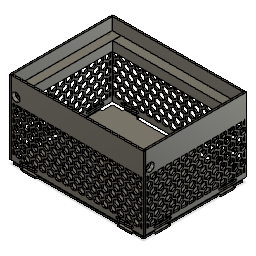
PSVR Storage Cube v1 (Autodesk Fusion 360 design; units mm, degrees)
Autodesk Fusion 360 part; units mm, degrees
(part 1 of 4)
sketch "Sketch1" plane through (0, 0, 0) normal (0, 1, 0) x (1, 0, 0)
  line L0 (0, 0) -> (151, 0)
  line L1 (151, 0) -> (151, 115)
  line L2 (151, 115) -> (0, 115)
  line L3 (0, 115) -> (0, 0)
  dimension "d1" = 151
  dimension "d2" = 115
  constraint horizontal L0
  constraint vertical L1
  constraint horizontal L2
  constraint vertical L3
  constraint coincident L0.start L3.end
  measures "d1" distance of L0.start L0.end
  measures "d2" distance of L0.start L2.end
extrude "Extrude1" add sketch "Sketch1" along normal blind 2 makes body 1
sketch "Sketch2" plane through (0, 0, 0) normal (0, 0, 1) x (1, 0, 0)
  line L0 (-150, 0) -> (1, 0)
  line L1 (1, 0) -> (1, 130)
  line L2 (1, 130) -> (-150, 130)
  line L3 (-150, 130) -> (-150, 0)
  line L4 (-150, 0) -> (1, 0)
  line L5 (1, 0) -> (1, 65)
  line L6 (1, 65) -> (-150, 65)
  line L7 (-150, 65) -> (-150, 0)
  dimension "d5" = 151
  dimension "d6" = 130
  dimension "d14" = 65
  constraint horizontal L0
  constraint vertical L1
  constraint horizontal L2
  constraint vertical L3
  constraint horizontal L4
  constraint vertical L5
  constraint horizontal L6
  constraint vertical L7
  measures "d5" distance of L0.start L0.end
  measures "d6" distance of L0.start L2.end
  measures "d14" distance of L0.start L6.end
extrude "Extrude2" add sketch "Sketch2" along normal blind 2 separate body contours L0 L1 L3 L4 L5 L6 L7 makes body 2
sketch "Sketch3" plane through (0, 0, 0) normal (1, 0, 0) x (0, 0, -1)
  line L0 (200, 0) -> (85, 0)
  line L1 (85, 0) -> (85, 130)
  line L2 (85, 130) -> (200, 130)
  line L3 (200, 130) -> (200, 0)
  line L4 (85, 0) -> (200, 0)
  line L5 (200, 0) -> (200, 65)
  line L6 (200, 65) -> (85, 65)
  line L7 (85, 65) -> (85, 0)
  dimension "d9" = 115
  dimension "d10" = 130
  dimension "d13" = 65
  constraint horizontal L0
  constraint vertical L1
  constraint horizontal L2
  constraint vertical L3
  constraint horizontal L4
  constraint vertical L5
  constraint horizontal L6
  constraint vertical L7
  measures "d9" distance of L0.start L0.end
  measures "d10" distance of L0.start L2.end
  measures "d13" distance of L0.end L6.end
extrude "Extrude3" add sketch "Sketch3" against normal blind 2 separate body contours L0 L1 L3 L4 L5 L6 L7 makes body 3
sketch "Sketch4" plane through (0, 0, 0) normal (1, 0, 0) x (0, 0, -1)
  line L0 (85, 0) -> (200, 0)
  line L1 (200, 0) -> (200, 65)
  line L2 (200, 65) -> (85, 65)
  line L3 (85, 65) -> (85, 0)
  line L4 (200, 0) -> (85, 0)
  line L5 (85, 0) -> (85, 40)
  line L6 (85, 40) -> (200, 40)
  line L7 (200, 40) -> (200, 0)
  line L8 (85, 40) -> (200, 40)
  line L9 (200, 40) -> (200, 51)
  line L10 (200, 51) -> (85, 51)
  line L11 (85, 51) -> (85, 40)
  line L12 (85, 40) -> (95.25, 40)
  line L13 (95.25, 40) -> (95.25, 51)
  line L14 (95.25, 51) -> (85, 51)
  line L15 (85, 51) -> (85, 40)
  dimension "d15" = 40
  dimension "d16" = 11
  dimension "d24" = 10.25
  constraint horizontal L4
  constraint vertical L5
  constraint horizontal L6
  constraint vertical L7
  constraint coincident L0.end L1.start
  constraint horizontal L8
  constraint vertical L9
  constraint horizontal L10
  constraint vertical L11
  constraint horizontal L12
  constraint vertical L13
  constraint horizontal L14
  constraint vertical L15
  measures "d15" distance of L0.end L6.end
  measures "d16" distance of L5.end L10.end
  measures "d24" distance of L5.end L12.end
extrude "Extrude4" add sketch "Sketch4" along normal blind 10 contours L1 L6 L8 L9 L10 L13 bodies 2 3 1
sketch "Sketch5" plane through (0, 0, 0) normal (0, 0, -1) x (-1, 0, 0)
  line L0 (-1, 0) -> (150, 0)
  line L1 (150, 0) -> (150, 65)
  line L2 (150, 65) -> (-1, 65)
  line L3 (-1, 65) -> (-1, 0)
  line L4 (150, 0) -> (-0.75, 0)
  line L5 (-0.75, 0) -> (-0.75, 40)
  line L6 (-0.75, 40) -> (150, 40)
  line L7 (150, 40) -> (150, 0)
  line L8 (-0.75, 40) -> (150, 40)
  line L9 (150, 40) -> (150, 51)
  line L10 (150, 51) -> (-0.75, 51)
  line L11 (-0.75, 51) -> (-0.75, 40)
  line L12 (-0.75, 40) -> (9.25, 40)
  line L13 (9.25, 40) -> (9.25, 51)
  line L14 (9.25, 51) -> (-0.75, 51)
  line L15 (-0.75, 51) -> (-0.75, 40)
  dimension "d19" = 40
  dimension "d20" = 11
  dimension "d23" = 10
  constraint horizontal L4
  constraint vertical L5
  constraint horizontal L6
  constraint vertical L7
  constraint coincident L0.end L1.start
  constraint horizontal L8
  constraint vertical L9
  constraint horizontal L10
  constraint vertical L11
  constraint horizontal L12
  constraint vertical L13
  constraint horizontal L14
  constraint vertical L15
  measures "d19" distance of L0.end L6.end
  measures "d20" distance of L5.end L10.end
  measures "d23" distance of L5.end L12.end
extrude "Extrude5" add sketch "Sketch5" along normal blind 10 contours L1 L6 L8 L9 L10 L13 bodies 3 1 2
extrude "Extrude6" add 1 faces at (-0.6667, 0, -161.6667) along direction (0, -1, 0) blind 20 on bodies 3 bodies 3
extrude "Extrude7" add 1 faces at (-99.6667, 0, 0.6667) along direction (0, -1, 0) blind 20 on bodies 2 bodies 2
move_body "Move1" bodies 2 to x (1, 0, 0) y (0, 1, 0) z (0, 0, 1) at (0, 20, 0)
move_body "Move2" bodies 3 to x (1, 0, 0) y (0, 1, 0) z (0, 0, 1) at (0, 22, 0)
move_body "Move3" bodies 2 to x (1, 0, 0) y (0, 1, 0) z (0, 0, 1) at (150, 0, 0)
move_body "Move4" bodies 3 to x (1, 0, 0) y (0, 1, 0) z (0, 0, 1) at (0, 0, 85)
move_body "Move5" bodies 3 to x (1, 0, 0) y (0, 1, 0) z (0, 0, 1) at (0, -2, 0)
extrude "Extrude8" add 1 faces at (151, 28.3333, 1.3333) along direction (1, 0, 0) blind 2 on bodies 2 bodies 2
extrude "Extrude9" add 1 faces at (-1.3333, 28.3333, 0) along direction (0, 0, 1) blind 2 on bodies 3 bodies 3
sketch "Sketch6" plane through (0, 0, 0) normal (0, 0, -1) x (-1, 0, 0)
  line L0 (-140.75, 71) -> (0, 71)
  line L1 (0, 71) -> (0, 85)
  line L2 (0, 85) -> (-153, 85)
  line L3 (-153, 85) -> (-153, 0)
  line L4 (-153, 0) -> (0, 0)
  line L5 (0, 0) -> (0, 60)
  line L6 (0, 60) -> (-140.75, 60)
  line L7 (-140.75, 60) -> (-140.75, 71)
  line L8 (-153, 0) -> (-141, 0)
  line L9 (-141, 0) -> (-141, 2)
  line L10 (-141, 2) -> (-153, 2)
  line L11 (-153, 2) -> (-153, 0)
  line L12 (-141, 2) -> (-121, 2)
  line L13 (-121, 2) -> (-121, 4.5)
  line L14 (-121, 4.5) -> (-141, 4.5)
  line L15 (-141, 4.5) -> (-141, 2)
  line L16 (0, 0) -> (-10, 0)
  line L17 (-10, 0) -> (-10, 2)
  line L18 (-10, 2) -> (0, 2)
  line L19 (0, 2) -> (0, 0)
  line L20 (-10, 2) -> (-30, 2)
  line L21 (-30, 2) -> (-30, 4.5)
  line L22 (-30, 4.5) -> (-10, 4.5)
  line L23 (-10, 4.5) -> (-10, 2)
  dimension "d33" = 12
  dimension "d34" = 2
  dimension "d35" = 20
  dimension "d36" = 2.5
  dimension "d37" = 10
  dimension "d38" = 2
  dimension "d39" = 20
  dimension "d40" = 2.5
  constraint horizontal L8
  constraint vertical L9
  constraint horizontal L10
  constraint vertical L11
  constraint coincident L3.end L4.start
  constraint horizontal L12
  constraint vertical L13
  constraint horizontal L14
  constraint vertical L15
  constraint horizontal L16
  constraint vertical L17
  constraint horizontal L18
  constraint vertical L19
  constraint coincident L4.end L5.start
  constraint horizontal L20
  constraint vertical L21
  constraint horizontal L22
  constraint vertical L23
  measures "d33" distance of L3.end L8.end
  measures "d34" distance of L3.end L10.end
  measures "d35" distance of L9.end L12.end
  measures "d36" distance of L9.end L14.end
  measures "d37" distance of L4.end L16.end
  measures "d38" distance of L4.end L18.end
  measures "d39" distance of L17.end L20.end
  measures "d40" distance of L17.end L22.end
extrude "Extrude10" cut sketch "Sketch6" against normal blind 2 contours L12 L13 L14 L15 | L20 L21 L22 L23 bodies 2
sketch "Sketch7" plane through (0, 0, 0) normal (1, 0, 0) x (0, 0, -1)
  line L0 (10.25, 71) -> (115, 71)
  line L1 (115, 71) -> (115, 85)
  line L2 (115, 85) -> (-2, 85)
  line L3 (-2, 85) -> (-2, 0)
  line L4 (-2, 0) -> (115, 0)
  line L5 (115, 0) -> (115, 60)
  line L6 (115, 60) -> (10.25, 60)
  line L7 (10.25, 60) -> (10.25, 71)
  line L8 (-2, 0) -> (10, 0)
  line L9 (10, 0) -> (10, 2)
  line L10 (10, 2) -> (-2, 2)
  line L11 (-2, 2) -> (-2, 0)
  line L12 (10, 2) -> (30, 2)
  line L13 (30, 2) -> (30, 4.5)
  line L14 (30, 4.5) -> (10, 4.5)
  line L15 (10, 4.5) -> (10, 2)
  line L16 (115, 0) -> (105, 0)
  line L17 (105, 0) -> (105, 2)
  line L18 (105, 2) -> (115, 2)
  line L19 (115, 2) -> (115, 0)
  line L20 (105, 2) -> (85, 2)
  line L21 (85, 2) -> (85, 4.5)
  line L22 (85, 4.5) -> (105, 4.5)
  line L23 (105, 4.5) -> (105, 2)
  dimension "d43" = 12
  dimension "d44" = 2
  dimension "d45" = 20
  dimension "d46" = 2.5
  dimension "d47" = 10
  dimension "d48" = 2
  dimension "d49" = 20
  dimension "d50" = 2.5
  constraint horizontal L8
  constraint vertical L9
  constraint horizontal L10
  constraint vertical L11
  constraint coincident L3.end L4.start
  constraint horizontal L12
  constraint vertical L13
  constraint horizontal L14
  constraint vertical L15
  constraint horizontal L16
  constraint vertical L17
  constraint horizontal L18
  constraint vertical L19
  constraint coincident L4.end L5.start
  constraint horizontal L20
  constraint vertical L21
  constraint horizontal L22
  constraint vertical L23
  measures "d43" distance of L3.end L8.end
  measures "d44" distance of L3.end L10.end
  measures "d45" distance of L9.end L12.end
  measures "d46" distance of L9.end L14.end
  measures "d47" distance of L4.end L16.end
  measures "d48" distance of L4.end L18.end
  measures "d49" distance of L17.end L20.end
  measures "d50" distance of L17.end L22.end
extrude "Extrude11" cut sketch "Sketch7" against normal blind 2 contours L12 L13 L14 L15 | L20 L21 L22 L23 bodies 3
move_body "Move6" bodies 1 to x (1, 0, 0) y (0, 1, 0) z (0, 0, 1) at (0, -5, 0)
sketch "Sketch8" plane through (0, -3, 0) normal (0, 1, 0) x (-1, 0, 0)
  line L0 (0, -115) -> (0, 0)
  line L1 (0, 0) -> (-151, 0)
  line L2 (-151, 0) -> (-151, -115)
  line L3 (-151, -115) -> (0, -115)
  line L4 (0, -115) -> (-20, -115)
  line L5 (-20, -115) -> (-29, -115)
  line L6 (-29, -115) -> (-11, -115)
  line L7 (-11, -115) -> (-11, -117)
  line L8 (-11, -117) -> (-29, -117)
  line L9 (-29, -117) -> (-29, -115)
  line L10 (-151, -115) -> (-122, -115)
  line L11 (-122, -115) -> (-140, -115)
  line L12 (-140, -115) -> (-140, -117)
  line L13 (-140, -117) -> (-122, -117)
  line L14 (-122, -117) -> (-122, -115)
  line L15 (0, -115) -> (0, -86)
  line L16 (0, -86) -> (2, -86)
  line L17 (2, -86) -> (2, -104)
  line L18 (2, -104) -> (0, -104)
  line L19 (0, -104) -> (0, -86)
  line L20 (-151, -115) -> (-151, -86)
  line L21 (-151, -86) -> (-153, -86)
  line L22 (-153, -86) -> (-153, -104)
  line L23 (-153, -104) -> (-151, -104)
  line L24 (-151, -104) -> (-151, -86)
  line L25 (-151, 0) -> (-122, 0)
  line L26 (-122, 0) -> (-140, 0)
  line L27 (-140, 0) -> (-140, 2)
  line L28 (-140, 2) -> (-122, 2)
  line L29 (-122, 2) -> (-122, 0)
  line L30 (-151, 0) -> (-151, -29)
  line L31 (-151, -29) -> (-153, -29)
  line L32 (-153, -29) -> (-153, -11)
  line L33 (-153, -11) -> (-151, -11)
  line L34 (-151, -11) -> (-151, -29)
  line L35 (0, 0) -> (-29, 0)
  line L36 (-29, 0) -> (-11, 0)
  line L37 (-11, 0) -> (-11, 2)
  line L38 (-11, 2) -> (-29, 2)
  line L39 (-29, 2) -> (-29, 0)
  line L40 (0, 0) -> (0, -29)
  line L41 (0, -29) -> (2, -29)
  line L42 (2, -29) -> (2, -11)
  line L43 (2, -11) -> (0, -11)
  line L44 (0, -11) -> (0, -29)
  dimension "d53" = 20
  dimension "d54" = 9
  dimension "d55" = 18
  dimension "d56" = 2
  dimension "d57" = 29
  dimension "d58" = 18
  dimension "d59" = 2
  dimension "d60" = 29
  dimension "d61" = 2
  dimension "d62" = 18
  dimension "d63" = 29
  dimension "d64" = 2
  dimension "d65" = 18
  dimension "d66" = 29
  dimension "d67" = 18
  dimension "d68" = 2
  dimension "d69" = 29
  dimension "d70" = 2
  dimension "d71" = 18
  dimension "d72" = 29
  dimension "d73" = 18
  dimension "d74" = 2
  dimension "d75" = 29
  dimension "d76" = 2
  dimension "d77" = 18
  constraint coincident L0.start L3.end
  constraint perpendicular L0 L4
  constraint parallel L3 L5
  constraint horizontal L6
  constraint vertical L7
  constraint horizontal L8
  constraint vertical L9
  constraint coincident L2.end L3.start
  constraint perpendicular L2 L10
  constraint horizontal L11
  constraint vertical L12
  constraint horizontal L13
  constraint vertical L14
  constraint perpendicular L4 L15
  constraint horizontal L16
  constraint vertical L17
  constraint horizontal L18
  constraint vertical L19
  constraint perpendicular L10 L20
  constraint horizontal L21
  constraint vertical L22
  constraint horizontal L23
  constraint vertical L24
  constraint coincident L1.end L2.start
  constraint perpendicular L2 L25
  constraint horizontal L26
  constraint vertical L27
  constraint horizontal L28
  constraint vertical L29
  constraint perpendicular L1 L30
  constraint horizontal L31
  constraint vertical L32
  constraint horizontal L33
  constraint vertical L34
  constraint coincident L0.end L1.start
  constraint perpendicular L0 L35
  constraint horizontal L36
  constraint vertical L37
  constraint horizontal L38
  constraint vertical L39
  constraint perpendicular L35 L40
  constraint horizontal L41
  constraint vertical L42
  constraint horizontal L43
  constraint vertical L44
  measures "d53" distance of L0.start L4.end
  measures "d54" distance of L4.end L5.end
  measures "d55" distance of L5.end L6.end
  measures "d56" distance of L5.end L8.end
  measures "d57" distance of L2.end L10.end
  measures "d58" distance of L10.end L11.end
  measures "d59" distance of L10.end L13.end
  measures "d60" distance of L0.start L15.end
  measures "d61" distance of L15.end L16.end
  measures "d62" distance of L15.end L18.end
  measures "d63" distance of L2.end L20.end
  measures "d64" distance of L20.end L21.end
  measures "d65" distance of L20.end L23.end
  measures "d66" distance of L1.end L25.end
  measures "d67" distance of L25.end L26.end
  measures "d68" distance of L25.end L28.end
  measures "d69" distance of L1.end L30.end
  measures "d70" distance of L30.end L31.end
  measures "d71" distance of L30.end L33.end
  measures "d72" distance of L0.end L35.end
  measures "d73" distance of L35.end L36.end
  measures "d74" distance of L35.end L38.end
  measures "d75" distance of L0.end L40.end
  measures "d76" distance of L40.end L41.end
  measures "d77" distance of L40.end L43.end
extrude "Extrude12" add sketch "Sketch8" against normal blind 2 contours L0 L15 L16 L17 L18 L19 | L3 L4 L5 L6 L7 L8 L9 | L0 L40 L41 L42 L43 L44 | L3 L10 L11 L12 L13 L14 | L1 L35 L36 L37 L38 L39 | L2 L20 L21 L22 L23 L24 | L1 L25 L26 L27 L28 L29 | L2 L30 L31 L32 L33 L34 bodies 1
fillet "Fillet1" radius 1 32 edges at (-1, -3, -11) (-1, -5, -11) (-1, -5, -29) (-1, -3, -29) (-1, -3, -104) (-1, -5, -104) (-1, -5, -86) (-1, -3, -86) (11, -3, -116) (11, -5, -116) (29, -3, -116) (29, -5, -116) (122, -3, -116) (140, -3, -116) (140, -5, -116) (152, -3, -104) (152, -5, -104) (152, -3, -86) (122, -5, -116) (152, -5, -86) (152, -3, -29) (152, -5, -29) (152, -3, -11) (152, -5, -11) (140, -5, 1) (140, -3, 1) (122, -5, 1) (122, -3, 1) (29, -3, 1) (29, -5, 1) (11, -3, 1) (11, -5, 1) on bodies 1
fillet "Fillet2" radius 1 16 edges at (141, 4.5, 1) (141, 2, 1) (30, 2, 1) (10, 2, 1) (10, 4.5, 1) (30, 4.5, 1) (121, 2, 1) (121, 4.5, 1) (-1, 4.5, -85) (-1, 4.5, -10) (-1, 2, -85) (-1, 2, -10) (-1, 4.5, -30) (-1, 2, -30) (-1, 2, -105) (-1, 4.5, -105) on bodies 2 3
move_face "OffsetFaces1" offset -0.25 12 faces at (151, -3.9049, -48) (151, -4.0001, -111.3333) (147.3333, -4.0001, -115) (91, -4.1159, -115) (151, -4.0001, -3.6667) (147.3333, -3.9999, 0) (60, -4.1159, 0) (3.6667, -4.0001, 0) (0, -4.0001, -3.6667) (0, -3.9049, -67) (0, -4.0001, -111.3333) (3.6667, -3.9999, -115) on bodies 1
sketch "Sketch9" plane through (0, 0, 0) normal (0, 0, -1) x (-1, 0, 0)
  line L0 (-30, 3) -> (-30, 3.5)
  arc A0 (-29, 4.5) -> (-30, 3.5) centre (-29, 3.5) ccw
  line L1 (-29, 4.5) -> (-11, 4.5)
  arc A1 (-10, 3.5) -> (-11, 4.5) centre (-11, 3.5) ccw
  line L2 (-10, 3.5) -> (-10, 3)
  arc A2 (-11, 2) -> (-10, 3) centre (-11, 3) ccw
  line L3 (-11, 2) -> (-29, 2)
  arc A3 (-30, 3) -> (-29, 2) centre (-29, 3) ccw
  line L4 (-122, 2) -> (-140, 2)
  arc A4 (-141, 3) -> (-140, 2) centre (-140, 3) ccw
  line L5 (-141, 3) -> (-141, 3.5)
  arc A5 (-140, 4.5) -> (-141, 3.5) centre (-140, 3.5) ccw
  line L6 (-140, 4.5) -> (-122, 4.5)
  arc A6 (-121, 3.5) -> (-122, 4.5) centre (-122, 3.5) ccw
  line L7 (-121, 3.5) -> (-121, 3)
  arc A7 (-122, 2) -> (-121, 3) centre (-122, 3) ccw
  line L8 (-140.75, 71) -> (0, 71)
  line L9 (0, 71) -> (0, 85)
  line L10 (0, 85) -> (-153, 85)
  line L11 (-153, 85) -> (-153, 0)
  line L12 (-153, 0) -> (0, 0)
  line L13 (0, 0) -> (0, 60)
  line L14 (0, 60) -> (-140.75, 60)
  line L15 (-140.75, 60) -> (-140.75, 71)
  line L16 (0, 60) -> (0, 71)
  line L17 (0, 65.5) -> (-5.5, 65.5)
  circle A8 centre (-5.5, 65.5) radius 4.75
  dimension "d85" = 5.5
  dimension "d86" = 9.5
  constraint coincident L13.end L14.start
  constraint coincident L8.end L9.start
  constraint midpoint L16 L17.start
  constraint perpendicular L16 L17
  constraint coincident L17.end A8.centre
  measures "d85" distance of L17.start L17.end
  measures "d86" diameter of A8
extrude "Extrude13" cut sketch "Sketch9" along normal blind 2 and the other way blind 2 contours A8 bodies 2
sketch "Sketch10" plane through (0, 0, -2) normal (0, 0, 1) x (1, 0, 0)
  circle A0 centre (5.5, 65.5) radius 4.75
  circle A1 centre (5.5, 65.5) radius 2.4
  dimension "d91" = 4.8
  constraint concentric A0 A1
  measures "d91" diameter of A1
extrude "Extrude14" cut sketch "Sketch10" against normal blind 25 contours A1 bodies 2 3
move_face "OffsetFaces2" offset -0.25 1 faces at (0, 67.3333, -6.6667) on bodies 2
sketch "Sketch11" plane through (0, 0, 0) normal (1, 0, 0) x (0, 0, -1)
  line L0 (85, 3) -> (85, 3.5)
  arc A0 (86, 4.5) -> (85, 3.5) centre (86, 3.5) ccw
  line L1 (86, 4.5) -> (104, 4.5)
  arc A1 (105, 3.5) -> (104, 4.5) centre (104, 3.5) ccw
  line L2 (105, 3.5) -> (105, 3)
  arc A2 (104, 2) -> (105, 3) centre (104, 3) ccw
  line L3 (104, 2) -> (86, 2)
  arc A3 (85, 3) -> (86, 2) centre (86, 3) ccw
  line L4 (29, 2) -> (11, 2)
  arc A4 (10, 3) -> (11, 2) centre (11, 3) ccw
  line L5 (10, 3) -> (10, 3.5)
  arc A5 (11, 4.5) -> (10, 3.5) centre (11, 3.5) ccw
  line L6 (11, 4.5) -> (29, 4.5)
  arc A6 (30, 3.5) -> (29, 4.5) centre (29, 3.5) ccw
  line L7 (30, 3.5) -> (30, 3)
  arc A7 (29, 2) -> (30, 3) centre (29, 3) ccw
  line L8 (10.25, 71) -> (115, 71)
  line L9 (115, 71) -> (115, 85)
  line L10 (115, 85) -> (-2, 85)
  line L11 (-2, 85) -> (-2, 0)
  line L12 (-2, 0) -> (115, 0)
  line L13 (115, 0) -> (115, 60)
  line L14 (115, 60) -> (10.25, 60)
  line L15 (10.25, 60) -> (10.25, 71)
  line L16 (115, 60) -> (115, 71)
  line L17 (115, 65.5) -> (109.5, 65.5)
  circle A8 centre (109.5, 65.5) radius 4.75
  dimension "d95" = 5.5
  dimension "d96" = 9.5
  constraint coincident L13.end L14.start
  constraint coincident L8.end L9.start
  constraint midpoint L16 L17.start
  constraint perpendicular L16 L17
  constraint coincident L17.end A8.centre
  measures "d95" distance of L17.start L17.end
  measures "d96" diameter of A8
extrude "Extrude15" cut sketch "Sketch11" along normal blind 2 and the other way blind 2 contours A8 bodies 3
sketch "Sketch12" plane through (2, 0, 0) normal (-1, 0, 0) x (0, 0, 1)
  circle A0 centre (-109.5, 65.5) radius 4.75
  circle A1 centre (-109.5, 65.5) radius 2.4
  dimension "d101" = 4.8
  constraint concentric A0 A1
  measures "d101" diameter of A1
extrude "Extrude16" cut sketch "Sketch12" against normal blind 33 contours A1 bodies 3
sketch "Sketch13" plane through (140.75, 0, 0) normal (1, 0, 0) x (0, 0, -1)
  line L0 (0, 71) -> (0, 60)
  line L1 (0, 60) -> (10, 60)
  line L2 (10, 60) -> (10, 71)
  line L3 (10, 71) -> (0, 71)
  line L4 (10, 65.5) -> (7.9, 65.5)
  circle A0 centre (5.5, 65.5) radius 2.4
  dimension "d104" = 2.1
  dimension "d105" = 4.8
  constraint midpoint L2 L4.start
  constraint perpendicular L2 L4
  constraint coincident L4.end A0
  measures "d104" distance of L4.start L4.end
  measures "d105" diameter of A0
extrude "Extrude17" cut sketch "Sketch13" against normal blind 16.75 contours A0 bodies 2
move_face "OffsetFaces3" offset -0.25 1 faces at (6.6667, 67.3333, -115) on bodies 3
sketch "Sketch14" plane through (0, 0, 0) normal (0, 0, -1) x (-1, 0, 0)
  line L0 (-30, 3) -> (-30, 3.5)
  arc A0 (-29, 4.5) -> (-30, 3.5) centre (-29, 3.5) ccw
  line L1 (-29, 4.5) -> (-11, 4.5)
  arc A1 (-10, 3.5) -> (-11, 4.5) centre (-11, 3.5) ccw
  line L2 (-10, 3.5) -> (-10, 3)
  arc A2 (-11, 2) -> (-10, 3) centre (-11, 3) ccw
  line L3 (-11, 2) -> (-29, 2)
  arc A3 (-30, 3) -> (-29, 2) centre (-29, 3) ccw
  line L4 (-122, 2) -> (-140, 2)
  arc A4 (-141, 3) -> (-140, 2) centre (-140, 3) ccw
  line L5 (-141, 3) -> (-141, 3.5)
  arc A5 (-140, 4.5) -> (-141, 3.5) centre (-140, 3.5) ccw
  line L6 (-140, 4.5) -> (-122, 4.5)
  arc A6 (-121, 3.5) -> (-122, 4.5) centre (-122, 3.5) ccw
  line L7 (-121, 3.5) -> (-121, 3)
  arc A7 (-122, 2) -> (-121, 3) centre (-122, 3) ccw
  line L8 (-140.75, 71) -> (-0.25, 71)
  line L9 (-0.25, 71) -> (-0.25, 85)
  line L10 (-0.25, 85) -> (-153, 85)
  line L11 (-153, 85) -> (-153, 0)
  line L12 (-153, 0) -> (-0.25, 0)
  line L13 (-0.25, 0) -> (-0.25, 60)
  line L14 (-0.25, 60) -> (-140.75, 60)
  line L15 (-140.75, 60) -> (-140.75, 71)
  line L16 (-153, 0) -> (-0.25, 0)
  line L17 (-0.25, 0) -> (-0.25, 6.5)
  line L18 (-0.25, 6.5) -> (-2.25, 6.5)
  line L19 (-2.25, 6.5) -> (-2.25, 85)
  line L20 (-2.25, 85) -> (-0.25, 85)
  line L21 (-0.25, 85) -> (-0.25, 6.5)
  line L22 (-2.25, 85) -> (-153, 85)
  line L23 (-153, 85) -> (-153, 83)
  line L24 (-153, 83) -> (-2.25, 83)
  line L25 (-2.25, 83) -> (-2.25, 85)
  line L26 (-153, 83) -> (-151, 83)
  line L27 (-151, 83) -> (-151, 6.5)
  line L28 (-153, 6.5) -> (-153, 83)
  line L29 (-2.25, 6.5) -> (-2.25, 60)
  line L30 (-2.25, 60) -> (-151, 60)
  line L31 (-151, 60) -> (-151, 6.5)
  line L32 (-153, 0) -> (-0.25, 0)
  line L33 (-0.25, 0) -> (-0.25, 7)
  line L34 (-0.25, 7) -> (-0.25, 0)
  line L35 (-0.25, 0) -> (-153, 0)
  line L36 (-153, 0) -> (-2.25, 0)
  line L37 (-2.25, 0) -> (-2.25, 6)
  line L38 (-2.25, 6) -> (-153, 6)
  line L39 (-153, 6) -> (-153, 0)
  line L40 (-151, 6.5) -> (-151, 6)
  line L41 (-73.125, 35.2707) -> (-76.625, 37.2915)
  line L42 (-76.625, 37.2915) -> (-80.125, 35.2707)
  line L43 (-80.125, 35.2707) -> (-80.125, 31.2293)
  line L44 (-80.125, 31.2293) -> (-76.625, 29.2085)
  line L45 (-76.625, 29.2085) -> (-73.125, 31.2293)
  line L46 (-73.125, 31.2293) -> (-73.125, 35.2707)
  line L47 (-64.125, 35.2707) -> (-67.625, 37.2915)
  line L48 (-67.625, 37.2915) -> (-71.125, 35.2707)
  line L49 (-71.125, 35.2707) -> (-71.125, 31.2293)
  line L50 (-71.125, 31.2293) -> (-67.625, 29.2085)
  line L51 (-67.625, 29.2085) -> (-64.125, 31.2293)
  line L52 (-64.125, 31.2293) -> (-64.125, 35.2707)
  line L53 (-68.625, 43.065) -> (-72.125, 45.0857)
  line L54 (-72.125, 45.0857) -> (-75.625, 43.065)
  line L55 (-75.625, 43.065) -> (-75.625, 39.0235)
  line L56 (-75.625, 39.0235) -> (-72.125, 37.0028)
  line L57 (-72.125, 37.0028) -> (-68.625, 39.0235)
  line L58 (-68.625, 39.0235) -> (-68.625, 43.065)
  line L59 (-77.625, 43.065) -> (-81.125, 45.0857)
  line L60 (-81.125, 45.0857) -> (-84.625, 43.065)
  line L61 (-84.625, 43.065) -> (-84.625, 39.0235)
  line L62 (-84.625, 39.0235) -> (-81.125, 37.0028)
  line L63 (-81.125, 37.0028) -> (-77.625, 39.0235)
  line L64 (-77.625, 39.0235) -> (-77.625, 43.065)
  line L65 (-140.625, 11.311) -> (-144.125, 13.3317)
  line L66 (-144.125, 13.3317) -> (-147.625, 11.311)
  line L67 (-140.625, 7.2695) -> (-140.625, 11.311)
  line L68 (-152.125, 3.5167) -> (-152.125, -0.5247)
  line L69 (-145.125, -0.5247) -> (-145.125, 3.5167)
  line L70 (-147.625, 7.2695) -> (-144.125, 5.2488)
  line L71 (-153.125, 13.3317) -> (-156.625, 11.311)
  line L72 (-149.625, 7.2695) -> (-149.625, 11.311)
  line L73 (-148.625, 5.5375) -> (-152.125, 3.5167)
  line L74 (-148.625, -2.5455) -> (-145.125, -0.5247)
  line L75 (-149.625, 11.311) -> (-153.125, 13.3317)
  line L76 (-156.625, 7.2695) -> (-153.125, 5.2488)
  line L77 (-153.125, 5.2488) -> (-149.625, 7.2695)
  line L78 (-145.125, 3.5167) -> (-148.625, 5.5375)
  line L79 (-147.625, 11.311) -> (-147.625, 7.2695)
  line L80 (-156.625, 11.311) -> (-156.625, 7.2695)
  line L81 (-144.125, 5.2488) -> (-140.625, 7.2695)
  line L82 (-139.625, 5.5375) -> (-143.125, 3.5167)
  line L83 (-136.125, 3.5167) -> (-139.625, 5.5375)
  line L84 (-139.625, -2.5455) -> (-136.125, -0.5247)
  line L85 (-143.125, 3.5167) -> (-143.125, -0.5247)
  line L86 (-143.125, -0.5247) -> (-139.625, -2.5455)
  line L87 (-136.125, -0.5247) -> (-136.125, 3.5167)
  line L88 (-152.125, -0.5247) -> (-148.625, -2.5455)
  line L89 (-122.625, 11.311) -> (-126.125, 13.3317)
  line L90 (-126.125, 13.3317) -> (-129.625, 11.311)
  line L91 (-122.625, 7.2695) -> (-122.625, 11.311)
  line L92 (-134.125, 3.5167) -> (-134.125, -0.5247)
  line L93 (-127.125, -0.5247) -> (-127.125, 3.5167)
  line L94 (-129.625, 7.2695) -> (-126.125, 5.2488)
  line L95 (-135.125, 13.3317) -> (-138.625, 11.311)
  line L96 (-131.625, 7.2695) -> (-131.625, 11.311)
  line L97 (-130.625, 5.5375) -> (-134.125, 3.5167)
  line L98 (-130.625, -2.5455) -> (-127.125, -0.5247)
  line L99 (-131.625, 11.311) -> (-135.125, 13.3317)
  line L100 (-138.625, 7.2695) -> (-135.125, 5.2488)
  line L101 (-135.125, 5.2488) -> (-131.625, 7.2695)
  line L102 (-127.125, 3.5167) -> (-130.625, 5.5375)
  line L103 (-129.625, 11.311) -> (-129.625, 7.2695)
  line L104 (-138.625, 11.311) -> (-138.625, 7.2695)
  line L105 (-126.125, 5.2488) -> (-122.625, 7.2695)
  line L106 (-121.625, 5.5375) -> (-125.125, 3.5167)
  line L107 (-118.125, 3.5167) -> (-121.625, 5.5375)
  line L108 (-121.625, -2.5455) -> (-118.125, -0.5247)
  line L109 (-125.125, 3.5167) -> (-125.125, -0.5247)
  line L110 (-125.125, -0.5247) -> (-121.625, -2.5455)
  line L111 (-118.125, -0.5247) -> (-118.125, 3.5167)
  line L112 (-134.125, -0.5247) -> (-130.625, -2.5455)
  line L113 (-104.625, 11.311) -> (-108.125, 13.3317)
  line L114 (-108.125, 13.3317) -> (-111.625, 11.311)
  line L115 (-104.625, 7.2695) -> (-104.625, 11.311)
  line L116 (-116.125, 3.5167) -> (-116.125, -0.5247)
  line L117 (-109.125, -0.5247) -> (-109.125, 3.5167)
  line L118 (-111.625, 7.2695) -> (-108.125, 5.2488)
  line L119 (-117.125, 13.3317) -> (-120.625, 11.311)
  line L120 (-113.625, 7.2695) -> (-113.625, 11.311)
  line L121 (-112.625, 5.5375) -> (-116.125, 3.5167)
  line L122 (-112.625, -2.5455) -> (-109.125, -0.5247)
  line L123 (-113.625, 11.311) -> (-117.125, 13.3317)
  line L124 (-120.625, 7.2695) -> (-117.125, 5.2488)
  line L125 (-117.125, 5.2488) -> (-113.625, 7.2695)
  line L126 (-109.125, 3.5167) -> (-112.625, 5.5375)
  line L127 (-111.625, 11.311) -> (-111.625, 7.2695)
  line L128 (-120.625, 11.311) -> (-120.625, 7.2695)
  line L129 (-108.125, 5.2488) -> (-104.625, 7.2695)
  line L130 (-103.625, 5.5375) -> (-107.125, 3.5167)
  line L131 (-100.125, 3.5167) -> (-103.625, 5.5375)
  line L132 (-103.625, -2.5455) -> (-100.125, -0.5247)
  line L133 (-107.125, 3.5167) -> (-107.125, -0.5247)
  line L134 (-107.125, -0.5247) -> (-103.625, -2.5455)
  line L135 (-100.125, -0.5247) -> (-100.125, 3.5167)
  line L136 (-116.125, -0.5247) -> (-112.625, -2.5455)
  line L137 (-86.625, 11.311) -> (-90.125, 13.3317)
  line L138 (-90.125, 13.3317) -> (-93.625, 11.311)
  line L139 (-86.625, 7.2695) -> (-86.625, 11.311)
  line L140 (-98.125, 3.5167) -> (-98.125, -0.5247)
  line L141 (-91.125, -0.5247) -> (-91.125, 3.5167)
  line L142 (-93.625, 7.2695) -> (-90.125, 5.2488)
  line L143 (-99.125, 13.3317) -> (-102.625, 11.311)
  line L144 (-95.625, 7.2695) -> (-95.625, 11.311)
  line L145 (-94.625, 5.5375) -> (-98.125, 3.5167)
  line L146 (-94.625, -2.5455) -> (-91.125, -0.5247)
  line L147 (-95.625, 11.311) -> (-99.125, 13.3317)
  line L148 (-102.625, 7.2695) -> (-99.125, 5.2488)
  line L149 (-99.125, 5.2488) -> (-95.625, 7.2695)
  line L150 (-91.125, 3.5167) -> (-94.625, 5.5375)
  line L151 (-93.625, 11.311) -> (-93.625, 7.2695)
  line L152 (-102.625, 11.311) -> (-102.625, 7.2695)
  line L153 (-90.125, 5.2488) -> (-86.625, 7.2695)
  line L154 (-85.625, 5.5375) -> (-89.125, 3.5167)
  line L155 (-82.125, 3.5167) -> (-85.625, 5.5375)
  line L156 (-85.625, -2.5455) -> (-82.125, -0.5247)
  line L157 (-89.125, 3.5167) -> (-89.125, -0.5247)
  line L158 (-89.125, -0.5247) -> (-85.625, -2.5455)
  line L159 (-82.125, -0.5247) -> (-82.125, 3.5167)
  line L160 (-98.125, -0.5247) -> (-94.625, -2.5455)
  line L161 (-68.625, 11.311) -> (-72.125, 13.3317)
  line L162 (-72.125, 13.3317) -> (-75.625, 11.311)
  line L163 (-68.625, 7.2695) -> (-68.625, 11.311)
  line L164 (-80.125, 3.5167) -> (-80.125, -0.5247)
  line L165 (-73.125, -0.5247) -> (-73.125, 3.5167)
  line L166 (-75.625, 7.2695) -> (-72.125, 5.2488)
  line L167 (-81.125, 13.3317) -> (-84.625, 11.311)
  line L168 (-77.625, 7.2695) -> (-77.625, 11.311)
  line L169 (-76.625, 5.5375) -> (-80.125, 3.5167)
  line L170 (-76.625, -2.5455) -> (-73.125, -0.5247)
  line L171 (-77.625, 11.311) -> (-81.125, 13.3317)
  line L172 (-84.625, 7.2695) -> (-81.125, 5.2488)
  line L173 (-81.125, 5.2488) -> (-77.625, 7.2695)
  line L174 (-73.125, 3.5167) -> (-76.625, 5.5375)
  line L175 (-75.625, 11.311) -> (-75.625, 7.2695)
  line L176 (-84.625, 11.311) -> (-84.625, 7.2695)
  line L177 (-72.125, 5.2488) -> (-68.625, 7.2695)
  line L178 (-67.625, 5.5375) -> (-71.125, 3.5167)
  line L179 (-64.125, 3.5167) -> (-67.625, 5.5375)
  line L180 (-67.625, -2.5455) -> (-64.125, -0.5247)
  line L181 (-71.125, 3.5167) -> (-71.125, -0.5247)
  line L182 (-71.125, -0.5247) -> (-67.625, -2.5455)
  line L183 (-64.125, -0.5247) -> (-64.125, 3.5167)
  line L184 (-80.125, -0.5247) -> (-76.625, -2.5455)
  line L185 (-50.625, 11.311) -> (-54.125, 13.3317)
  line L186 (-54.125, 13.3317) -> (-57.625, 11.311)
  line L187 (-50.625, 7.2695) -> (-50.625, 11.311)
  line L188 (-62.125, 3.5167) -> (-62.125, -0.5247)
  line L189 (-55.125, -0.5247) -> (-55.125, 3.5167)
  line L190 (-57.625, 7.2695) -> (-54.125, 5.2488)
  line L191 (-63.125, 13.3317) -> (-66.625, 11.311)
  line L192 (-59.625, 7.2695) -> (-59.625, 11.311)
  line L193 (-58.625, 5.5375) -> (-62.125, 3.5167)
  line L194 (-58.625, -2.5455) -> (-55.125, -0.5247)
  line L195 (-59.625, 11.311) -> (-63.125, 13.3317)
  line L196 (-66.625, 7.2695) -> (-63.125, 5.2488)
  line L197 (-63.125, 5.2488) -> (-59.625, 7.2695)
  line L198 (-55.125, 3.5167) -> (-58.625, 5.5375)
  line L199 (-57.625, 11.311) -> (-57.625, 7.2695)
  line L200 (-66.625, 11.311) -> (-66.625, 7.2695)
  line L201 (-54.125, 5.2488) -> (-50.625, 7.2695)
  line L202 (-49.625, 5.5375) -> (-53.125, 3.5167)
  line L203 (-46.125, 3.5167) -> (-49.625, 5.5375)
  line L204 (-49.625, -2.5455) -> (-46.125, -0.5247)
  line L205 (-53.125, 3.5167) -> (-53.125, -0.5247)
  line L206 (-53.125, -0.5247) -> (-49.625, -2.5455)
  line L207 (-46.125, -0.5247) -> (-46.125, 3.5167)
  line L208 (-62.125, -0.5247) -> (-58.625, -2.5455)
  line L209 (-32.625, 11.311) -> (-36.125, 13.3317)
  line L210 (-36.125, 13.3317) -> (-39.625, 11.311)
  line L211 (-32.625, 7.2695) -> (-32.625, 11.311)
  line L212 (-44.125, 3.5167) -> (-44.125, -0.5247)
  line L213 (-37.125, -0.5247) -> (-37.125, 3.5167)
  line L214 (-39.625, 7.2695) -> (-36.125, 5.2488)
  line L215 (-45.125, 13.3317) -> (-48.625, 11.311)
  line L216 (-41.625, 7.2695) -> (-41.625, 11.311)
  line L217 (-40.625, 5.5375) -> (-44.125, 3.5167)
  line L218 (-40.625, -2.5455) -> (-37.125, -0.5247)
  line L219 (-41.625, 11.311) -> (-45.125, 13.3317)
  line L220 (-48.625, 7.2695) -> (-45.125, 5.2488)
  line L221 (-45.125, 5.2488) -> (-41.625, 7.2695)
  line L222 (-37.125, 3.5167) -> (-40.625, 5.5375)
  line L223 (-39.625, 11.311) -> (-39.625, 7.2695)
  line L224 (-48.625, 11.311) -> (-48.625, 7.2695)
  line L225 (-36.125, 5.2488) -> (-32.625, 7.2695)
  line L226 (-31.625, 5.5375) -> (-35.125, 3.5167)
  line L227 (-28.125, 3.5167) -> (-31.625, 5.5375)
  line L228 (-31.625, -2.5455) -> (-28.125, -0.5247)
  line L229 (-35.125, 3.5167) -> (-35.125, -0.5247)
  line L230 (-35.125, -0.5247) -> (-31.625, -2.5455)
  line L231 (-28.125, -0.5247) -> (-28.125, 3.5167)
  line L232 (-44.125, -0.5247) -> (-40.625, -2.5455)
  line L233 (-14.625, 11.311) -> (-18.125, 13.3317)
  line L234 (-18.125, 13.3317) -> (-21.625, 11.311)
  line L235 (-14.625, 7.2695) -> (-14.625, 11.311)
  line L236 (-26.125, 3.5167) -> (-26.125, -0.5247)
  line L237 (-19.125, -0.5247) -> (-19.125, 3.5167)
  line L238 (-21.625, 7.2695) -> (-18.125, 5.2488)
  line L239 (-27.125, 13.3317) -> (-30.625, 11.311)
  line L240 (-23.625, 7.2695) -> (-23.625, 11.311)
  line L241 (-22.625, 5.5375) -> (-26.125, 3.5167)
  line L242 (-22.625, -2.5455) -> (-19.125, -0.5247)
  line L243 (-23.625, 11.311) -> (-27.125, 13.3317)
  line L244 (-30.625, 7.2695) -> (-27.125, 5.2488)
  line L245 (-27.125, 5.2488) -> (-23.625, 7.2695)
  line L246 (-19.125, 3.5167) -> (-22.625, 5.5375)
  line L247 (-21.625, 11.311) -> (-21.625, 7.2695)
  line L248 (-30.625, 11.311) -> (-30.625, 7.2695)
  line L249 (-18.125, 5.2488) -> (-14.625, 7.2695)
  line L250 (-13.625, 5.5375) -> (-17.125, 3.5167)
  line L251 (-10.125, 3.5167) -> (-13.625, 5.5375)
  line L252 (-13.625, -2.5455) -> (-10.125, -0.5247)
  line L253 (-17.125, 3.5167) -> (-17.125, -0.5247)
  line L254 (-17.125, -0.5247) -> (-13.625, -2.5455)
  line L255 (-10.125, -0.5247) -> (-10.125, 3.5167)
  line L256 (-26.125, -0.5247) -> (-22.625, -2.5455)
  line L257 (3.375, 11.311) -> (-0.125, 13.3317)
  line L258 (-0.125, 13.3317) -> (-3.625, 11.311)
  line L259 (3.375, 7.2695) -> (3.375, 11.311)
  line L260 (-8.125, 3.5167) -> (-8.125, -0.5247)
  line L261 (-1.125, -0.5247) -> (-1.125, 3.5167)
  line L262 (-3.625, 7.2695) -> (-0.125, 5.2488)
  line L263 (-9.125, 13.3317) -> (-12.625, 11.311)
  line L264 (-5.625, 7.2695) -> (-5.625, 11.311)
  line L265 (-4.625, 5.5375) -> (-8.125, 3.5167)
  line L266 (-4.625, -2.5455) -> (-1.125, -0.5247)
  line L267 (-5.625, 11.311) -> (-9.125, 13.3317)
  line L268 (-12.625, 7.2695) -> (-9.125, 5.2488)
  line L269 (-9.125, 5.2488) -> (-5.625, 7.2695)
  line L270 (-1.125, 3.5167) -> (-4.625, 5.5375)
  line L271 (-3.625, 11.311) -> (-3.625, 7.2695)
  line L272 (-12.625, 11.311) -> (-12.625, 7.2695)
  line L273 (-0.125, 5.2488) -> (3.375, 7.2695)
  line L274 (4.375, 5.5375) -> (0.875, 3.5167)
  line L275 (7.875, 3.5167) -> (4.375, 5.5375)
  line L276 (4.375, -2.5455) -> (7.875, -0.5247)
  line L277 (0.875, 3.5167) -> (0.875, -0.5247)
  line L278 (0.875, -0.5247) -> (4.375, -2.5455)
  line L279 (7.875, -0.5247) -> (7.875, 3.5167)
  line L280 (-8.125, -0.5247) -> (-4.625, -2.5455)
  line L281 (21.375, 11.311) -> (17.875, 13.3317)
  line L282 (17.875, 13.3317) -> (14.375, 11.311)
  line L283 (21.375, 7.2695) -> (21.375, 11.311)
  line L284 (9.875, 3.5167) -> (9.875, -0.5247)
  line L285 (16.875, -0.5247) -> (16.875, 3.5167)
  line L286 (14.375, 7.2695) -> (17.875, 5.2488)
  line L287 (8.875, 13.3317) -> (5.375, 11.311)
  line L288 (12.375, 7.2695) -> (12.375, 11.311)
  line L289 (13.375, 5.5375) -> (9.875, 3.5167)
  line L290 (13.375, -2.5455) -> (16.875, -0.5247)
  line L291 (12.375, 11.311) -> (8.875, 13.3317)
  line L292 (5.375, 7.2695) -> (8.875, 5.2488)
  line L293 (8.875, 5.2488) -> (12.375, 7.2695)
  line L294 (16.875, 3.5167) -> (13.375, 5.5375)
  line L295 (14.375, 11.311) -> (14.375, 7.2695)
  line L296 (5.375, 11.311) -> (5.375, 7.2695)
  line L297 (17.875, 5.2488) -> (21.375, 7.2695)
  line L298 (22.375, 5.5375) -> (18.875, 3.5167)
  line L299 (25.875, 3.5167) -> (22.375, 5.5375)
  line L300 (22.375, -2.5455) -> (25.875, -0.5247)
  line L301 (18.875, 3.5167) -> (18.875, -0.5247)
  line L302 (18.875, -0.5247) -> (22.375, -2.5455)
  line L303 (25.875, -0.5247) -> (25.875, 3.5167)
  line L304 (9.875, -0.5247) -> (13.375, -2.5455)
  line L305 (-140.625, 27.188) -> (-144.125, 29.2087)
  line L306 (-144.125, 29.2087) -> (-147.625, 27.188)
  line L307 (-140.625, 23.1465) -> (-140.625, 27.188)
  line L308 (-152.125, 19.3937) -> (-152.125, 15.3523)
  line L309 (-145.125, 15.3523) -> (-145.125, 19.3937)
  line L310 (-147.625, 23.1465) -> (-144.125, 21.1258)
  line L311 (-153.125, 29.2087) -> (-156.625, 27.188)
  line L312 (-149.625, 23.1465) -> (-149.625, 27.188)
  line L313 (-148.625, 21.4145) -> (-152.125, 19.3937)
  line L314 (-148.625, 13.3315) -> (-145.125, 15.3523)
  line L315 (-149.625, 27.188) -> (-153.125, 29.2087)
  line L316 (-156.625, 23.1465) -> (-153.125, 21.1258)
  line L317 (-153.125, 21.1258) -> (-149.625, 23.1465)
  line L318 (-145.125, 19.3937) -> (-148.625, 21.4145)
  line L319 (-147.625, 27.188) -> (-147.625, 23.1465)
  line L320 (-156.625, 27.188) -> (-156.625, 23.1465)
  line L321 (-144.125, 21.1258) -> (-140.625, 23.1465)
  line L322 (-139.625, 21.4145) -> (-143.125, 19.3937)
  line L323 (-136.125, 19.3937) -> (-139.625, 21.4145)
  line L324 (-139.625, 13.3315) -> (-136.125, 15.3523)
  line L325 (-143.125, 19.3937) -> (-143.125, 15.3523)
  line L326 (-143.125, 15.3523) -> (-139.625, 13.3315)
  line L327 (-136.125, 15.3523) -> (-136.125, 19.3937)
  line L328 (-152.125, 15.3523) -> (-148.625, 13.3315)
  line L329 (-122.625, 27.188) -> (-126.125, 29.2087)
  line L330 (-126.125, 29.2087) -> (-129.625, 27.188)
  line L331 (-122.625, 23.1465) -> (-122.625, 27.188)
  line L332 (-134.125, 19.3937) -> (-134.125, 15.3523)
  line L333 (-127.125, 15.3523) -> (-127.125, 19.3937)
  line L334 (-129.625, 23.1465) -> (-126.125, 21.1258)
  line L335 (-135.125, 29.2087) -> (-138.625, 27.188)
  line L336 (-131.625, 23.1465) -> (-131.625, 27.188)
  line L337 (-130.625, 21.4145) -> (-134.125, 19.3937)
  line L338 (-130.625, 13.3315) -> (-127.125, 15.3523)
  line L339 (-131.625, 27.188) -> (-135.125, 29.2087)
  line L340 (-138.625, 23.1465) -> (-135.125, 21.1258)
  line L341 (-135.125, 21.1258) -> (-131.625, 23.1465)
  line L342 (-127.125, 19.3937) -> (-130.625, 21.4145)
  line L343 (-129.625, 27.188) -> (-129.625, 23.1465)
  line L344 (-138.625, 27.188) -> (-138.625, 23.1465)
  line L345 (-126.125, 21.1258) -> (-122.625, 23.1465)
  line L346 (-121.625, 21.4145) -> (-125.125, 19.3937)
  line L347 (-118.125, 19.3937) -> (-121.625, 21.4145)
  line L348 (-121.625, 13.3315) -> (-118.125, 15.3523)
  line L349 (-125.125, 19.3937) -> (-125.125, 15.3523)
  line L350 (-125.125, 15.3523) -> (-121.625, 13.3315)
  line L351 (-118.125, 15.3523) -> (-118.125, 19.3937)
  line L352 (-134.125, 15.3523) -> (-130.625, 13.3315)
  line L353 (-104.625, 27.188) -> (-108.125, 29.2087)
  line L354 (-108.125, 29.2087) -> (-111.625, 27.188)
  line L355 (-104.625, 23.1465) -> (-104.625, 27.188)
  line L356 (-116.125, 19.3937) -> (-116.125, 15.3523)
  line L357 (-109.125, 15.3523) -> (-109.125, 19.3937)
  line L358 (-111.625, 23.1465) -> (-108.125, 21.1258)
  line L359 (-117.125, 29.2087) -> (-120.625, 27.188)
  line L360 (-113.625, 23.1465) -> (-113.625, 27.188)
  line L361 (-112.625, 21.4145) -> (-116.125, 19.3937)
  line L362 (-112.625, 13.3315) -> (-109.125, 15.3523)
  line L363 (-113.625, 27.188) -> (-117.125, 29.2087)
  line L364 (-120.625, 23.1465) -> (-117.125, 21.1258)
  line L365 (-117.125, 21.1258) -> (-113.625, 23.1465)
  line L366 (-109.125, 19.3937) -> (-112.625, 21.4145)
  line L367 (-111.625, 27.188) -> (-111.625, 23.1465)
  line L368 (-120.625, 27.188) -> (-120.625, 23.1465)
  line L369 (-108.125, 21.1258) -> (-104.625, 23.1465)
  line L370 (-103.625, 21.4145) -> (-107.125, 19.3937)
  line L371 (-100.125, 19.3937) -> (-103.625, 21.4145)
  line L372 (-103.625, 13.3315) -> (-100.125, 15.3523)
  line L373 (-107.125, 19.3937) -> (-107.125, 15.3523)
  line L374 (-107.125, 15.3523) -> (-103.625, 13.3315)
  line L375 (-100.125, 15.3523) -> (-100.125, 19.3937)
  line L376 (-116.125, 15.3523) -> (-112.625, 13.3315)
  line L377 (-86.625, 27.188) -> (-90.125, 29.2087)
  line L378 (-90.125, 29.2087) -> (-93.625, 27.188)
  line L379 (-86.625, 23.1465) -> (-86.625, 27.188)
  line L380 (-98.125, 19.3937) -> (-98.125, 15.3523)
  line L381 (-91.125, 15.3523) -> (-91.125, 19.3937)
  line L382 (-93.625, 23.1465) -> (-90.125, 21.1258)
  line L383 (-99.125, 29.2087) -> (-102.625, 27.188)
  line L384 (-95.625, 23.1465) -> (-95.625, 27.188)
  line L385 (-94.625, 21.4145) -> (-98.125, 19.3937)
  line L386 (-94.625, 13.3315) -> (-91.125, 15.3523)
  line L387 (-95.625, 27.188) -> (-99.125, 29.2087)
  line L388 (-102.625, 23.1465) -> (-99.125, 21.1258)
  line L389 (-99.125, 21.1258) -> (-95.625, 23.1465)
  line L390 (-91.125, 19.3937) -> (-94.625, 21.4145)
  line L391 (-93.625, 27.188) -> (-93.625, 23.1465)
  line L392 (-102.625, 27.188) -> (-102.625, 23.1465)
  line L393 (-90.125, 21.1258) -> (-86.625, 23.1465)
  line L394 (-85.625, 21.4145) -> (-89.125, 19.3937)
  line L395 (-82.125, 19.3937) -> (-85.625, 21.4145)
  line L396 (-85.625, 13.3315) -> (-82.125, 15.3523)
  line L397 (-89.125, 19.3937) -> (-89.125, 15.3523)
  line L398 (-89.125, 15.3523) -> (-85.625, 13.3315)
  line L399 (-82.125, 15.3523) -> (-82.125, 19.3937)
  line L400 (-98.125, 15.3523) -> (-94.625, 13.3315)
  line L401 (-68.625, 27.188) -> (-72.125, 29.2087)
  line L402 (-72.125, 29.2087) -> (-75.625, 27.188)
  line L403 (-68.625, 23.1465) -> (-68.625, 27.188)
  line L404 (-80.125, 19.3937) -> (-80.125, 15.3523)
  line L405 (-73.125, 15.3523) -> (-73.125, 19.3937)
  line L406 (-75.625, 23.1465) -> (-72.125, 21.1258)
  line L407 (-81.125, 29.2087) -> (-84.625, 27.188)
  line L408 (-77.625, 23.1465) -> (-77.625, 27.188)
  line L409 (-76.625, 21.4145) -> (-80.125, 19.3937)
  line L410 (-76.625, 13.3315) -> (-73.125, 15.3523)
  line L411 (-77.625, 27.188) -> (-81.125, 29.2087)
  line L412 (-84.625, 23.1465) -> (-81.125, 21.1258)
  line L413 (-81.125, 21.1258) -> (-77.625, 23.1465)
  line L414 (-73.125, 19.3937) -> (-76.625, 21.4145)
  line L415 (-75.625, 27.188) -> (-75.625, 23.1465)
  line L416 (-84.625, 27.188) -> (-84.625, 23.1465)
  line L417 (-72.125, 21.1258) -> (-68.625, 23.1465)
  line L418 (-67.625, 21.4145) -> (-71.125, 19.3937)
  line L419 (-64.125, 19.3937) -> (-67.625, 21.4145)
  line L420 (-67.625, 13.3315) -> (-64.125, 15.3523)
  line L421 (-71.125, 19.3937) -> (-71.125, 15.3523)
  line L422 (-71.125, 15.3523) -> (-67.625, 13.3315)
  line L423 (-64.125, 15.3523) -> (-64.125, 19.3937)
  line L424 (-80.125, 15.3523) -> (-76.625, 13.3315)
  line L425 (-50.625, 27.188) -> (-54.125, 29.2087)
  line L426 (-54.125, 29.2087) -> (-57.625, 27.188)
  line L427 (-50.625, 23.1465) -> (-50.625, 27.188)
  line L428 (-62.125, 19.3937) -> (-62.125, 15.3523)
  line L429 (-55.125, 15.3523) -> (-55.125, 19.3937)
  line L430 (-57.625, 23.1465) -> (-54.125, 21.1258)
  line L431 (-63.125, 29.2087) -> (-66.625, 27.188)
  line L432 (-59.625, 23.1465) -> (-59.625, 27.188)
  line L433 (-58.625, 21.4145) -> (-62.125, 19.3937)
  line L434 (-58.625, 13.3315) -> (-55.125, 15.3523)
  line L435 (-59.625, 27.188) -> (-63.125, 29.2087)
  line L436 (-66.625, 23.1465) -> (-63.125, 21.1258)
  line L437 (-63.125, 21.1258) -> (-59.625, 23.1465)
  line L438 (-55.125, 19.3937) -> (-58.625, 21.4145)
  line L439 (-57.625, 27.188) -> (-57.625, 23.1465)
  line L440 (-66.625, 27.188) -> (-66.625, 23.1465)
  line L441 (-54.125, 21.1258) -> (-50.625, 23.1465)
  line L442 (-49.625, 21.4145) -> (-53.125, 19.3937)
  line L443 (-46.125, 19.3937) -> (-49.625, 21.4145)
  line L444 (-49.625, 13.3315) -> (-46.125, 15.3523)
  line L445 (-53.125, 19.3937) -> (-53.125, 15.3523)
  line L446 (-53.125, 15.3523) -> (-49.625, 13.3315)
  line L447 (-46.125, 15.3523) -> (-46.125, 19.3937)
  line L448 (-62.125, 15.3523) -> (-58.625, 13.3315)
  line L449 (-32.625, 27.188) -> (-36.125, 29.2087)
  line L450 (-36.125, 29.2087) -> (-39.625, 27.188)
  line L451 (-32.625, 23.1465) -> (-32.625, 27.188)
  line L452 (-44.125, 19.3937) -> (-44.125, 15.3523)
  line L453 (-37.125, 15.3523) -> (-37.125, 19.3937)
  line L454 (-39.625, 23.1465) -> (-36.125, 21.1258)
  line L455 (-45.125, 29.2087) -> (-48.625, 27.188)
  line L456 (-41.625, 23.1465) -> (-41.625, 27.188)
  line L457 (-40.625, 21.4145) -> (-44.125, 19.3937)
  line L458 (-40.625, 13.3315) -> (-37.125, 15.3523)
  line L459 (-41.625, 27.188) -> (-45.125, 29.2087)
  line L460 (-48.625, 23.1465) -> (-45.125, 21.1258)
  line L461 (-45.125, 21.1258) -> (-41.625, 23.1465)
  line L462 (-37.125, 19.3937) -> (-40.625, 21.4145)
  line L463 (-39.625, 27.188) -> (-39.625, 23.1465)
  line L464 (-48.625, 27.188) -> (-48.625, 23.1465)
  line L465 (-36.125, 21.1258) -> (-32.625, 23.1465)
  line L466 (-31.625, 21.4145) -> (-35.125, 19.3937)
  line L467 (-28.125, 19.3937) -> (-31.625, 21.4145)
  line L468 (-31.625, 13.3315) -> (-28.125, 15.3523)
  line L469 (-35.125, 19.3937) -> (-35.125, 15.3523)
  line L470 (-35.125, 15.3523) -> (-31.625, 13.3315)
  line L471 (-28.125, 15.3523) -> (-28.125, 19.3937)
  line L472 (-44.125, 15.3523) -> (-40.625, 13.3315)
  line L473 (-14.625, 27.188) -> (-18.125, 29.2087)
  line L474 (-18.125, 29.2087) -> (-21.625, 27.188)
  line L475 (-14.625, 23.1465) -> (-14.625, 27.188)
  line L476 (-26.125, 19.3937) -> (-26.125, 15.3523)
  line L477 (-19.125, 15.3523) -> (-19.125, 19.3937)
  line L478 (-21.625, 23.1465) -> (-18.125, 21.1258)
  line L479 (-27.125, 29.2087) -> (-30.625, 27.188)
  line L480 (-23.625, 23.1465) -> (-23.625, 27.188)
  line L481 (-22.625, 21.4145) -> (-26.125, 19.3937)
  line L482 (-22.625, 13.3315) -> (-19.125, 15.3523)
  line L483 (-23.625, 27.188) -> (-27.125, 29.2087)
  line L484 (-30.625, 23.1465) -> (-27.125, 21.1258)
  line L485 (-27.125, 21.1258) -> (-23.625, 23.1465)
  line L486 (-19.125, 19.3937) -> (-22.625, 21.4145)
  line L487 (-21.625, 27.188) -> (-21.625, 23.1465)
  line L488 (-30.625, 27.188) -> (-30.625, 23.1465)
  line L489 (-18.125, 21.1258) -> (-14.625, 23.1465)
  line L490 (-13.625, 21.4145) -> (-17.125, 19.3937)
  line L491 (-10.125, 19.3937) -> (-13.625, 21.4145)
  line L492 (-13.625, 13.3315) -> (-10.125, 15.3523)
  line L493 (-17.125, 19.3937) -> (-17.125, 15.3523)
  line L494 (-17.125, 15.3523) -> (-13.625, 13.3315)
  line L495 (-10.125, 15.3523) -> (-10.125, 19.3937)
  line L496 (-26.125, 15.3523) -> (-22.625, 13.3315)
  line L497 (3.375, 27.188) -> (-0.125, 29.2087)
  line L498 (-0.125, 29.2087) -> (-3.625, 27.188)
  line L499 (3.375, 23.1465) -> (3.375, 27.188)
  line L500 (-8.125, 19.3937) -> (-8.125, 15.3523)
  line L501 (-1.125, 15.3523) -> (-1.125, 19.3937)
  line L502 (-3.625, 23.1465) -> (-0.125, 21.1258)
  line L503 (-9.125, 29.2087) -> (-12.625, 27.188)
  line L504 (-5.625, 23.1465) -> (-5.625, 27.188)
  line L505 (-4.625, 21.4145) -> (-8.125, 19.3937)
  line L506 (-4.625, 13.3315) -> (-1.125, 15.3523)
  line L507 (-5.625, 27.188) -> (-9.125, 29.2087)
  line L508 (-12.625, 23.1465) -> (-9.125, 21.1258)
  line L509 (-9.125, 21.1258) -> (-5.625, 23.1465)
  line L510 (-1.125, 19.3937) -> (-4.625, 21.4145)
  line L511 (-3.625, 27.188) -> (-3.625, 23.1465)
  line L512 (-12.625, 27.188) -> (-12.625, 23.1465)
  line L513 (-0.125, 21.1258) -> (3.375, 23.1465)
  line L514 (4.375, 21.4145) -> (0.875, 19.3937)
  line L515 (7.875, 19.3937) -> (4.375, 21.4145)
  line L516 (4.375, 13.3315) -> (7.875, 15.3523)
  line L517 (0.875, 19.3937) -> (0.875, 15.3523)
  line L518 (0.875, 15.3523) -> (4.375, 13.3315)
  line L519 (7.875, 15.3523) -> (7.875, 19.3937)
  line L520 (-8.125, 15.3523) -> (-4.625, 13.3315)
  line L521 (21.375, 27.188) -> (17.875, 29.2087)
  line L522 (17.875, 29.2087) -> (14.375, 27.188)
  line L523 (21.375, 23.1465) -> (21.375, 27.188)
  line L524 (9.875, 19.3937) -> (9.875, 15.3523)
  line L525 (16.875, 15.3523) -> (16.875, 19.3937)
  line L526 (14.375, 23.1465) -> (17.875, 21.1258)
  line L527 (8.875, 29.2087) -> (5.375, 27.188)
  line L528 (12.375, 23.1465) -> (12.375, 27.188)
  line L529 (13.375, 21.4145) -> (9.875, 19.3937)
  line L530 (13.375, 13.3315) -> (16.875, 15.3523)
  line L531 (12.375, 27.188) -> (8.875, 29.2087)
  line L532 (5.375, 23.1465) -> (8.875, 21.1258)
  line L533 (8.875, 21.1258) -> (12.375, 23.1465)
  line L534 (16.875, 19.3937) -> (13.375, 21.4145)
  line L535 (14.375, 27.188) -> (14.375, 23.1465)
  line L536 (5.375, 27.188) -> (5.375, 23.1465)
  line L537 (17.875, 21.1258) -> (21.375, 23.1465)
  line L538 (22.375, 21.4145) -> (18.875, 19.3937)
  line L539 (25.875, 19.3937) -> (22.375, 21.4145)
  line L540 (22.375, 13.3315) -> (25.875, 15.3523)
  line L541 (18.875, 19.3937) -> (18.875, 15.3523)
  line L542 (18.875, 15.3523) -> (22.375, 13.3315)
  line L543 (25.875, 15.3523) -> (25.875, 19.3937)
  line L544 (9.875, 15.3523) -> (13.375, 13.3315)
  line L545 (-140.625, 43.065) -> (-144.125, 45.0857)
  line L546 (-144.125, 45.0857) -> (-147.625, 43.065)
  line L547 (-140.625, 39.0235) -> (-140.625, 43.065)
  line L548 (-152.125, 35.2707) -> (-152.125, 31.2293)
  line L549 (-145.125, 31.2293) -> (-145.125, 35.2707)
  line L550 (-147.625, 39.0235) -> (-144.125, 37.0028)
  line L551 (-153.125, 45.0857) -> (-156.625, 43.065)
  line L552 (-149.625, 39.0235) -> (-149.625, 43.065)
  line L553 (-148.625, 37.2915) -> (-152.125, 35.2707)
  line L554 (-148.625, 29.2085) -> (-145.125, 31.2293)
  line L555 (-149.625, 43.065) -> (-153.125, 45.0857)
  line L556 (-156.625, 39.0235) -> (-153.125, 37.0028)
  line L557 (-153.125, 37.0028) -> (-149.625, 39.0235)
  line L558 (-145.125, 35.2707) -> (-148.625, 37.2915)
  line L559 (-147.625, 43.065) -> (-147.625, 39.0235)
  line L560 (-156.625, 43.065) -> (-156.625, 39.0235)
  line L561 (-144.125, 37.0028) -> (-140.625, 39.0235)
  line L562 (-139.625, 37.2915) -> (-143.125, 35.2707)
  line L563 (-136.125, 35.2707) -> (-139.625, 37.2915)
  line L564 (-139.625, 29.2085) -> (-136.125, 31.2293)